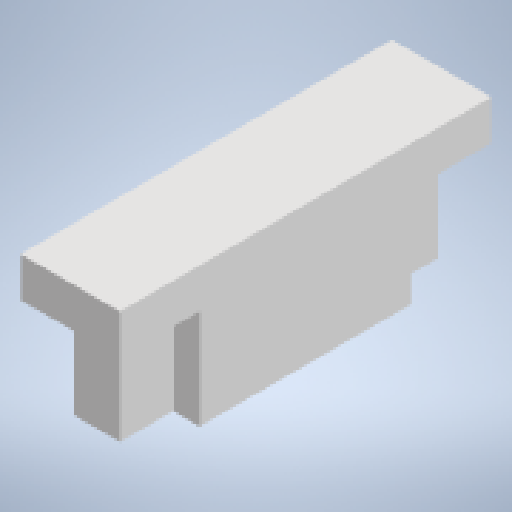
# Autodesk Inventor part: Connector
Saved by Autodesk Inventor 2023 (Build 270158000, 158)
## iProperties
Created: 2023-02-18
Part Number: Connector
Material: Generic
Document SubType Name: Modeling
Designer: phill
Density: 1 g/cm^3
Appearance: Default
Author: phill
Autodesk Inventor part; units mm, degrees
ref_plane "YZ Plane" through (0, 0, 0) normal (1, 0, 0) x (0, 1, 0)
ref_plane "XZ Plane" through (0, 0, 0) normal (0, 1, 0) x (-1, 0, 0)
ref_plane "XY Plane" through (0, 0, 0) normal (0, 0, 1) x (1, 0, 0)
sketch "Sketch1" plane through (0, 0, 0) normal (0, 1, 0) x (-1, 0, 0)
  line L0 (4, 4) -> (11, 4) projected
  line L1 (11, -8) -> (4, -8) projected
  line L2 (11, -52) -> (4, -52) projected
  line L3 (4, -40) -> (11, -40) projected
  line L4 (15, -8) -> (0, -8)
  line L5 (0, -8) -> (0, -40)
  line L6 (0, -40) -> (15, -40)
  line L7 (15, -40) -> (15, -8)
  line L8 (11, 4) -> (11, -8) projected
  line L9 (4, 4) -> (4, -8) projected
  line L10 (4, -52) -> (4, -40) projected
  line L11 (11, -52) -> (11, -40) projected
  point P0 (4, 0)
  point P1 (11, 0)
  point P2 (11, -48)
  point P3 (4, -48)
  point P4 (0, -8)
  point P5 (15, -40)
  constraints: 8 end point, 2 parallel, 1 horizontal, 1 perpendicular
extrude "Extrusion1" add sketch "Sketch1" against normal blind 15
sketch "Sketch2" plane through (0, 0, 0) normal (0, 1, 0) x (1, 0, 0)
  line L0 (-4, 8) -> (0, 8) projected
  line L1 (0, 8) -> (0, 40) projected
  line L2 (0, 40) -> (-4, 40) projected
  line L3 (-11, 40) -> (-15, 40) projected
  line L4 (-15, 40) -> (-15, 8) projected
  line L5 (-15, 8) -> (-11, 8) projected
  line L6 (-11, 52) -> (-4, 52) projected
  line L7 (-4, 40) -> (-11, 40) projected
  line L8 (-4, -4) -> (-11, -4) projected
  line L9 (-11, 8) -> (-4, 8) projected
  line L10 (-11, 52) -> (-11, 40) projected
  line L11 (-11, 8) -> (-11, -4) projected
  line L12 (-11, -4) -> (-4, -4) projected
  line L13 (-4, -4) -> (-4, 8) projected
  line L14 (-4, 40) -> (-4, 52) projected
  line L15 (-4, 52) -> (-11, 52) projected
  line L16 (-4, 52) -> (-4, 40) projected
  line L17 (-11, 52) -> (-11, 40) projected
  line L18 (-11, -4) -> (-11, 8) projected
  line L19 (-4, -4) -> (-4, 8) projected
  point P0 (-4, 0)
  point P1 (-4, 48)
  point P2 (-11, 48)
  point P3 (-11, 0)
extrude "Extrusion2" add sketch "Sketch2" along normal blind 6
sketch "Sketch3" plane through (0, 0, -52) normal (0, 0, -1) x (-1, 0, 0)
  line L0 (4, 6) -> (11, 6) projected
  line L1 (11, -15) -> (4, -15) projected
  line L2 (11, 6) -> (11, -15) projected
  line L3 (4, -15) -> (4, 6) projected
  point P0 (0, 0)
body "Solid1"
